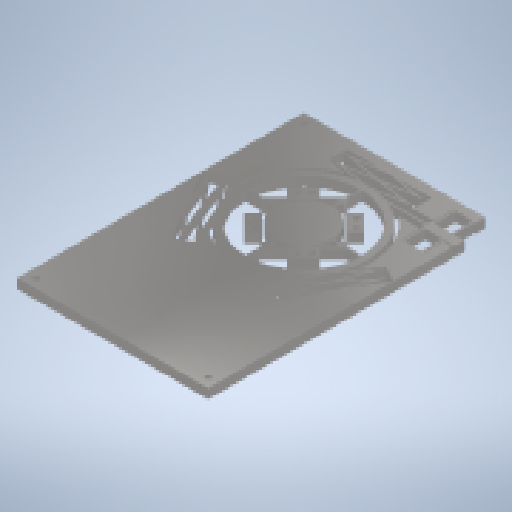
# Autodesk Inventor part: FlexBloc
Saved by Autodesk Inventor 2023 (Build 270158000, 158)
## iProperties
Created: 2023-03-17
Part Number: FlexBloc
Material: Steel, Mild
Document SubType Name: Modeling
Designer: Nathann
Density: 7.85 g/cm^3
Appearance: Semi-Polished
Mass: 505.648 g
Surface Area: 323.574 cm^2
Volume: 64.4137 cm^3
Author: Nathann
Autodesk Inventor part; units mm, degrees
ref_plane "YZ Plane" through (0, 0, 0) normal (1, 0, 0) x (0, 1, 0)
ref_plane "XZ Plane" through (0, 0, 0) normal (0, 1, 0) x (-1, 0, 0)
ref_plane "XY Plane" through (0, 0, 0) normal (0, 0, 1) x (1, 0, 0)
sketch "Sketch1" plane through (0, 0, 0) normal (0, 1, 0) x (-1, 0, 0)
  line L0 (0, 0) -> (100, 0)
  line L1 (100, 0) -> (100, 150)
  line L2 (100, 150) -> (0, 150)
  line L3 (0, 150) -> (0, 0)
  dimension "d0" = 150
  dimension "d1" = 100
  constraints: 8 end point, 2 parallel, 1 horizontal, 1 perpendicular
  measures "d0" distance of L2.end L0.start
  measures "d1" distance of L0.start L0.end
extrude "Extrusion1" add sketch "Sketch1" along normal blind 5
sketch "Sketch6" plane through (0, 5, 0) normal (0, 1, 0) x (1, 0, 0)
  circle A0 centre (-50, -50) radius 15
  line L0 (0, -150) -> (0, 0) projected
  line L1 (0, 0) -> (-100, 0) projected
  circle A1 centre (-50, -50) radius 30
  circle A2 centre (-50, -50) radius 33.541
  line L2 (-64.4545, -50.5) -> (-85.4944, -50.5)
  line L3 (-85.4944, -50.5) -> (-85.4944, -49.5)
  line L4 (-85.4944, -49.5) -> (-64.4545, -49.5)
  line L5 (-64.4545, -49.5) -> (-64.4545, -50.5)
  line L6 (-50, -50) -> (-59.276, -50)
  circle A3 centre (-50, -50) radius 36.041
  line L7 (-65, -50) -> (-80, -50)
  line L8 (-67.5, -50) -> (-70, -52.5)
  line L9 (-67.5, -50) -> (-70, -47.5)
  line L10 (-70, -52.5) -> (-70.7463, -51.7537)
  line L11 (-70, -47.5) -> (-74.2837, -51.7837)
  line L12 (-70, -52.5) -> (-72.5, -50)
  line L13 (-72.5, -50) -> (-70, -47.5)
  line L14 (-73.2071, -50) -> (-70.3536, -52.8536)
  line L15 (-70.3536, -52.8536) -> (-70, -52.5)
  line L16 (-73.2071, -50) -> (-70.3536, -47.1464)
  line L17 (-70.3536, -47.1464) -> (-70, -47.5)
  line L18 (-70.3536, -52.8536) -> (-65.8462, -57.3609)
  line L19 (-65.8462, -57.3609) -> (-65.1391, -56.6538)
  line L20 (-65.1391, -56.6538) -> (-69.6464, -52.1464)
  line L21 (-70.3536, -47.1464) -> (-65.8462, -42.6391)
  line L22 (-65.8462, -42.6391) -> (-65.1391, -43.3462)
  line L23 (-65.1391, -43.3462) -> (-69.6464, -47.8536)
  line L24 (-50, -50) -> (-54.8166, -54.8166)
  line L25 (-50, -50) -> (-57.7269, -42.2731)
  line L26 (-65.1391, -56.6538) -> (-70.0888, -61.6036)
  line L27 (-70.0888, -61.6036) -> (-65.8462, -65.8462)
  line L28 (-65.8462, -65.8462) -> (-60.8964, -60.8964)
  line L29 (-60.8964, -60.8964) -> (-65.1391, -56.6538)
  circle A4 centre (-65.8462, -61.6036) radius 1.5
  line L30 (-64.4545, -50) -> (-69.6304, -50)
  line L31 (-65.1391, -43.3462) -> (-70.0888, -38.3964)
  line L32 (-70.0888, -38.3964) -> (-65.8462, -34.1538)
  line L33 (-65.8462, -34.1538) -> (-60.8964, -39.1036)
  line L34 (-60.8964, -39.1036) -> (-65.1391, -43.3462)
  circle A5 centre (-65.8462, -38.3964) radius 1.5
  line L35 (-50, -64.4545) -> (-50, -69.6304)
  line L36 (-34.1538, -65.8462) -> (-39.1036, -60.8964)
  line L37 (-39.1036, -60.8964) -> (-43.3462, -65.1391)
  line L38 (-42.6391, -65.8462) -> (-43.3462, -65.1391)
  circle A6 centre (-38.3964, -65.8462) radius 1.5
  line L39 (-43.3462, -65.1391) -> (-38.3964, -70.0888)
  line L40 (-50, -67.5) -> (-52.5, -70)
  line L41 (-50, -67.5) -> (-47.5, -70)
  line L42 (-47.1464, -70.3536) -> (-42.6391, -65.8462)
  line L43 (-49.5, -64.4545) -> (-49.5, -85.4944)
  line L44 (-43.3462, -65.1391) -> (-47.8536, -69.6464)
  line L45 (-50.5, -85.4944) -> (-50.5, -64.4545)
  line L46 (-47.5, -70) -> (-48.2463, -70.7463)
  line L47 (-49.5, -85.4944) -> (-50.5, -85.4944)
  line L48 (-38.3964, -70.0888) -> (-34.1538, -65.8462)
  line L49 (-50.5, -64.4545) -> (-49.5, -64.4545)
  line L50 (-50, -65) -> (-50, -80)
  line L51 (-47.1464, -70.3536) -> (-47.5, -70)
  line L52 (-52.8536, -70.3536) -> (-52.5, -70)
  line L53 (-47.5, -70) -> (-50, -72.5)
  line L54 (-50, -73.2071) -> (-47.1464, -70.3536)
  line L55 (-50, -72.5) -> (-52.5, -70)
  line L56 (-50, -73.2071) -> (-52.8536, -70.3536)
  line L57 (-52.5, -70) -> (-48.2163, -74.2837)
  line L58 (-56.6538, -65.1391) -> (-52.1464, -69.6464)
  line L59 (-52.8536, -70.3536) -> (-57.3609, -65.8462)
  line L60 (-60.8964, -60.8964) -> (-56.6538, -65.1391)
  line L61 (-56.6538, -65.1391) -> (-61.6036, -70.0888)
  circle A7 centre (-61.6036, -65.8462) radius 1.5
  line L62 (-65.8462, -65.8462) -> (-60.8964, -60.8964)
  line L63 (-61.6036, -70.0888) -> (-65.8462, -65.8462)
  line L64 (-57.3609, -65.8462) -> (-56.6538, -65.1391)
  line L65 (-35.5455, -50) -> (-30.3696, -50)
  line L66 (-34.1538, -34.1538) -> (-39.1036, -39.1036)
  line L67 (-39.1036, -39.1036) -> (-34.8609, -43.3462)
  line L68 (-34.1538, -42.6391) -> (-34.8609, -43.3462)
  circle A8 centre (-34.1538, -38.3964) radius 1.5
  line L69 (-34.8609, -43.3462) -> (-29.9112, -38.3964)
  line L70 (-32.5, -50) -> (-30, -52.5)
  line L71 (-32.5, -50) -> (-30, -47.5)
  line L72 (-29.6464, -47.1464) -> (-34.1538, -42.6391)
  line L73 (-35.5455, -49.5) -> (-14.5056, -49.5)
  line L74 (-34.8609, -43.3462) -> (-30.3536, -47.8536)
  line L75 (-14.5056, -50.5) -> (-35.5455, -50.5)
  line L76 (-30, -47.5) -> (-29.2537, -48.2463)
  line L77 (-14.5056, -49.5) -> (-14.5056, -50.5)
  line L78 (-29.9112, -38.3964) -> (-34.1538, -34.1538)
  line L79 (-35.5455, -50.5) -> (-35.5455, -49.5)
  line L80 (-35, -50) -> (-20, -50)
  line L81 (-29.6464, -47.1464) -> (-30, -47.5)
  line L82 (-29.6464, -52.8536) -> (-30, -52.5)
  line L83 (-30, -47.5) -> (-27.5, -50)
  line L84 (-26.7929, -50) -> (-29.6464, -47.1464)
  line L85 (-27.5, -50) -> (-30, -52.5)
  line L86 (-26.7929, -50) -> (-29.6464, -52.8536)
  line L87 (-30, -52.5) -> (-25.7163, -48.2163)
  line L88 (-34.8609, -56.6538) -> (-30.3536, -52.1464)
  line L89 (-29.6464, -52.8536) -> (-34.1538, -57.3609)
  line L90 (-39.1036, -60.8964) -> (-34.8609, -56.6538)
  line L91 (-34.8609, -56.6538) -> (-29.9112, -61.6036)
  circle A9 centre (-34.1538, -61.6036) radius 1.5
  line L92 (-34.1538, -65.8462) -> (-39.1036, -60.8964)
  line L93 (-29.9112, -61.6036) -> (-34.1538, -65.8462)
  line L94 (-34.1538, -57.3609) -> (-34.8609, -56.6538)
  line L95 (-50, -35.5455) -> (-50, -30.3696)
  line L96 (-65.8462, -34.1538) -> (-60.8964, -39.1036)
  line L97 (-60.8964, -39.1036) -> (-56.6538, -34.8609)
  line L98 (-57.3609, -34.1538) -> (-56.6538, -34.8609)
  circle A10 centre (-61.6036, -34.1538) radius 1.5
  line L99 (-56.6538, -34.8609) -> (-61.6036, -29.9112)
  line L100 (-50, -32.5) -> (-47.5, -30)
  line L101 (-50, -32.5) -> (-52.5, -30)
  line L102 (-52.8536, -29.6464) -> (-57.3609, -34.1538)
  line L103 (-50.5, -35.5455) -> (-50.5, -14.5056)
  line L104 (-56.6538, -34.8609) -> (-52.1464, -30.3536)
  line L105 (-49.5, -14.5056) -> (-49.5, -35.5455)
  line L106 (-52.5, -30) -> (-51.7537, -29.2537)
  line L107 (-50.5, -14.5056) -> (-49.5, -14.5056)
  line L108 (-61.6036, -29.9112) -> (-65.8462, -34.1538)
  line L109 (-49.5, -35.5455) -> (-50.5, -35.5455)
  line L110 (-50, -35) -> (-50, -20)
  line L111 (-52.8536, -29.6464) -> (-52.5, -30)
  line L112 (-47.1464, -29.6464) -> (-47.5, -30)
  line L113 (-52.5, -30) -> (-50, -27.5)
  line L114 (-50, -26.7929) -> (-52.8536, -29.6464)
  line L115 (-50, -27.5) -> (-47.5, -30)
  line L116 (-50, -26.7929) -> (-47.1464, -29.6464)
  line L117 (-47.5, -30) -> (-51.7837, -25.7163)
  line L118 (-43.3462, -34.8609) -> (-47.8536, -30.3536)
  line L119 (-47.1464, -29.6464) -> (-42.6391, -34.1538)
  line L120 (-39.1036, -39.1036) -> (-43.3462, -34.8609)
  line L121 (-43.3462, -34.8609) -> (-38.3964, -29.9112)
  circle A11 centre (-38.3964, -34.1538) radius 1.5
  line L122 (-34.1538, -34.1538) -> (-39.1036, -39.1036)
  line L123 (-38.3964, -29.9112) -> (-34.1538, -34.1538)
  line L124 (-42.6391, -34.1538) -> (-43.3462, -34.8609)
  point P0 (-67.9675, -36.2751)
  point P1 (-63.7249, -67.9675)
  point P2 (-32.0325, -63.7249)
  point P3 (-36.2751, -32.0325)
  point P4 (-49.5, -72.7071)
  point P5 (-49.5, -79.9958)
  point P6 (-20.0042, -50.5)
  point P7 (-27.2929, -50.5)
  point P8 (-34.1538, -42.6391)
  point P9 (-27.2929, -49.5)
  point P10 (-20.0042, -49.5)
  point P11 (-49.5, -20.0042)
  point P12 (-49.5, -27.2929)
  point P13 (-68, -49.5)
  point P14 (-64.9917, -49.5)
  point P15 (-50.5, -35.0083)
  point P16 (-50.5, -32)
  point P17 (-49.5, -32)
  point P18 (-49.5, -35.0083)
  point P19 (-35.0083, -49.5)
  point P20 (-32, -49.5)
  point P21 (-32, -50.5)
  point P22 (-35.0083, -50.5)
  point P23 (-49.5, -64.9917)
  point P24 (-49.5, -68)
  point P25 (-50.5, -68)
  point P26 (-50.5, -64.9917)
  point P27 (-64.9917, -50.5)
  point P28 (-68, -50.5)
  point P29 (-57.3609, -34.1538)
  point P30 (-50.5, -27.2929)
  point P31 (-50.5, -20.0042)
  point P32 (-79.9958, -49.5)
  point P33 (-72.7071, -49.5)
  point P34 (-72.7071, -50.5)
  point P35 (-79.9958, -50.5)
  point P36 (-50.5, -79.9958)
  point P37 (-50.5, -72.7071)
  point P38 (-83.5373, -50.5)
  point P39 (-83.5373, -49.5)
  point P40 (-50.5, -16.4627)
  point P41 (-49.5, -16.4627)
  point P42 (-16.4627, -49.5)
  point P43 (-16.4627, -50.5)
  point P44 (-49.5, -83.5373)
  point P45 (-50.5, -83.5373)
  dimension "d80" = 30
  dimension "d81" = 60
  dimension "d78" = 50
  dimension "d79" = 50
  dimension "d82" = 67.082
  dimension "d83" = 0.5
  dimension "d84" = 0.5
  dimension "d91" = 72.082
  dimension "d92" = 5
  dimension "d93" = 2.5
  dimension "d94" = 2.5
  dimension "d95" = 45
  dimension "d96" = 45
  dimension "d97" = 0.5
  dimension "d98" = 0.5
  dimension "d99" = 0.5
  dimension "d100" = 45
  dimension "d101" = 45
  dimension "d102" = 6
  dimension "d103" = 7
  dimension "d104" = 3
  dimension "d105" = 3
  dimension "d106" = 3
  dimension "d107" = 3
  dimension "d108" = 7.5
  dimension "d109" = 3
  dimension "d110" = 6
  dimension "d111" = 7
  dimension "d112" = 3
  dimension "d113" = 3
  dimension "d114" = 3
  dimension "d117" = 360
  constraints: 246 end point, 20 point on line, 15 perpendicular, 10 centre point, 9 parallel, 3 coincident, 3 horizontal, 3 midpoint, 264 other
  measures "d78" distance from line of point (-50, -50) L0
  measures "d79" distance from line of L1 point (-50, -50)
  measures "d82" diameter of A2
  measures "d83" distance between parallel lines of L4 L6
  measures "d84" distance from line of point (-50, -50) L2
  measures "d91" diameter of A3
  measures "d92" distance of L8.start L12.end
  measures "d93" horizontal distance of L12.end L9.end
  measures "d94" horizontal distance of L8.end L12.end
  measures "d95" angle of L7 L8
  measures "d96" angle of L9 L7
  measures "d97" distance of L14.end L8.end
  measures "d98" distance between parallel lines of L10 L20
  measures "d99" distance between parallel lines of L23 L11
  measures "d100" angle of L24 L6
  measures "d101" angle of L25 L6
  measures "d102" distance of L28.end L19.end
  measures "d103" distance of L19.end L26.end
  measures "d104" distance from line of L27 A4.centre
  measures "d105" distance from line of L26 A4.centre
  measures "d106" diameter of A4
  measures "d107" distance from line of L24 A4.centre
  measures "d108" distance of L7.start L12.end
  measures "d109" distance of point (-67.968, -36.275) A5.centre
  measures "d110" distance of L33.end L22.end
  measures "d111" distance of L32.end L33.end
  measures "d112" distance from line of L33 A5.centre
  measures "d113" diameter of A5
  measures "d114" distance from line of A5.centre L25
extrude "Extrusion6" cut sketch "Sketch6" against normal blind 10 contours A0 L105 L100 L118 L120 L67 L74 L71 L73 | L75 L70 L88 L90 L37 L44 L41 L43 A0 | A0 L4 L9 L23 L34 L97 L104 L101 L103 | L84 L72 L69 L78 L123 L121 L119 L116 L105 A1 L73 | L45 L40 L58 L60 L29 L20 L8 L2 A0 | L75 A1 L43 L54 L42 L39 L48 L93 L91 L89 L86 | A2 L73 L77 L75 | L114 L102 L99 L108 L32 L31 L21 L16 L4 A1 L103 | A2 L103 L107 L105 | L45 A1 L2 L14 L18 L26 L27 L63 L61 L59 L56 | L43 L47 L45 A2 | A2 L2 L3 L4 | A4 | A5 | A6 | A7 | A8 | A9 | A10 | A11
sketch "Sketch7" plane through (0, 5, 0) normal (0, 1, 0) x (1, 0, 0)
  line L0 (-30.2515, -22) -> (6.5047, -22)
  line L1 (6.5047, -22) -> (6.5047, -15)
  line L2 (6.5047, -15) -> (-23.9617, -15)
  line L3 (-50, -60) -> (-28.7023, -38.7023)
  line L4 (-50, -60) -> (0, -60)
  line L5 (-11.682, -22) -> (-5.682, -22)
  line L6 (-2.365, -15) -> (-8.365, -15)
  line L7 (-5, -22) -> (-17, -22)
  line L8 (-17, -22) -> (-17, -32)
  line L9 (-17, -32) -> (-5, -32)
  line L10 (-5, -32) -> (-5, -22)
  line L11 (-5, -15) -> (-17, -15)
  line L12 (-17, -15) -> (-17, -5)
  line L13 (-17, -5) -> (-5, -5)
  line L14 (-5, -5) -> (-5, -15)
  line L15 (0, 0) -> (-100, 0) projected
  line L16 (0, -150) -> (0, 0) projected
  line L17 (-16.5, -32) -> (-15.5, -32)
  line L18 (-15.5, -32) -> (-15.5, -21)
  line L19 (-15.5, -21) -> (-16.5, -21)
  line L20 (-16.5, -21) -> (-16.5, -32)
  line L21 (-5.5, -32) -> (-6.5, -32)
  line L22 (-6.5, -32) -> (-6.5, -21)
  line L23 (-6.5, -21) -> (-5.5, -21)
  line L24 (-5.5, -21) -> (-5.5, -32)
  line L25 (-5.5, -5) -> (-6.5, -5)
  line L26 (-6.5, -5) -> (-6.5, -16)
  line L27 (-6.5, -16) -> (-5.5, -16)
  line L28 (-5.5, -16) -> (-5.5, -5)
  line L29 (-16.5, -5) -> (-15.5, -5)
  line L30 (-15.5, -5) -> (-15.5, -16)
  line L31 (-15.5, -16) -> (-16.5, -16)
  line L32 (-16.5, -16) -> (-16.5, -5)
  line L33 (-17.539, -21) -> (0, -21)
  line L34 (0, -21) -> (0, -16)
  line L35 (0, -16) -> (-17.539, -16)
  arc A0 (-49.5, -16.4627) -> (-50.5, -16.4627) centre (-50, -50) ccw projected
  line L36 (0, 0) -> (-5, 0)
  line L37 (-5, 0) -> (-5, -16)
  line L38 (-5, -16) -> (0, -16)
  line L39 (0, -16) -> (0, 0)
  line L40 (-17.539, -21) -> (-17.539, -16)
  line L41 (-20.9617, -19) -> (-17.539, -19)
  line L42 (-17.539, -19) -> (-17.539, -18)
  line L43 (-17.539, -18) -> (-20.9617, -18)
  line L44 (-23.9617, -15) -> (-23.9617, -22)
  line L45 (-23.9617, -22) -> (-30.2515, -22)
  line L46 (-20.9617, -18) -> (-20.9617, -19)
  point P0 (-5.5, -10.5)
  point P1 (-5, -27)
  point P2 (-16, -21)
  point P3 (-16, -16)
  point P4 (-17, -15)
  point P5 (-17, -22)
  point P6 (-15.5, -5)
  point P7 (-15.5, -16)
  point P8 (-6.5, -16)
  point P9 (-6.5, -5)
  point P10 (-5.5, -16)
  point P11 (0, -16)
  point P12 (0, -15)
  point P13 (0, -21)
  point P14 (0, -22)
  point P15 (-6.5, -32)
  point P16 (-5, -5)
  point P17 (-15.5, -15)
  point P18 (-16.5, -15)
  point P19 (-15.5, -22)
  point P20 (-16.5, -22)
  point P21 (-16.5, -15)
  point P22 (-16.5, -22)
  point P23 (-6.5, -22)
  point P24 (-15.5, -22)
  point P25 (-5.5, -22)
  point P26 (-5.5, -15)
  point P27 (-15.5, -15)
  point P28 (-6.5, -15)
  dimension "d125" = 45
  dimension "d128" = 10
  dimension "d133" = 12
  dimension "d134" = 12
  dimension "d135" = 5
  dimension "d136" = 1
  dimension "d137" = 1
  dimension "d138" = 1
  dimension "d139" = 1
  dimension "d140" = 0.5
  dimension "d141" = 0.5
  dimension "d142" = 11
  dimension "d144" = 11
  dimension "d145" = 11
  dimension "d146" = 10
  dimension "d147" = 11
  dimension "d164" = 5
  dimension "d169" = 0
  dimension "d170" = 5
  dimension "d171" = 1
  dimension "d172" = 2
  dimension "d202" = 5
  dimension "d214" = 3
  constraints: 90 end point, 17 parallel, 17 point on line, 13 horizontal, 12 perpendicular, 4 midpoint, 2 vertical
  measures "d125" angle of L3 L4
  measures "d128" distance of L9.end L7.start
  measures "d133" distance of L8.end L9.end
  measures "d134" distance of L12.end L13.end
  measures "d135" distance between parallel lines of L16 L10
  measures "d136" distance between parallel lines of L18 L20
  measures "d137" distance between parallel lines of L22 L24
  measures "d138" distance from line of L26 point (-5.5, -10.5)
  measures "d139" distance between parallel lines of L32 L30
  measures "d140" distance between parallel lines of L8 L20
  measures "d141" distance from line of point (-5, -27) L24
  measures "d142" distance of L17.end L18.end
  measures "d144" distance of L29.end L30.end
  measures "d145" distance of L27.end L25.start
  measures "d146" distance of L11.end L12.end
  measures "d147" distance of L21.end L22.end
  measures "d164" distance between parallel lines of L16 L37
  measures "d169" distance between parallel lines of L34 L16
  measures "d170" distance between parallel lines of L35 L33
  measures "d171" distance between parallel lines of L43 L41
  measures "d172" distance between parallel lines of L35 L43
  measures "d202" distance between parallel lines of L15 L13
  measures "d214" distance between parallel lines of L46 L44
extrude "Extrusion7" cut sketch "Sketch7" against normal blind 5 contours L44 L2 L32 L35 L40 L43 L46 L41 L33 L20 L0 | L0 L20 L9 L8 | L12 L13 L32 L2 | L18 L33 L22 L0 | L0 L22 L9 L18 | L30 L13 L26 L2 | L2 L26 L35 L30 | L24 L0 L10 L9 | L33 L16 L0 L24 | L16 L2 L1 L0 | L28 L13 L14 L2 | L2 L37 L35 L28 | L35 L37 L2 L16 | L14 L37 L15 L16 L2
sketch "Sketch9" plane through (0, 5, 0) normal (0, 1, 0) x (1, 0, 0)
  arc A0 (-35.0083, -49.5) -> (-49.5, -35.0083) centre (-50, -50) ccw projected
  line L0 (-50, -50) -> (-50, -7.3451)
  arc A1 (-49.5, -16.4627) -> (-50.5, -16.4627) centre (-50, -50) ccw projected
  line L1 (-50, -16.459) -> (-35, -13.959)
  line L2 (-35, -13.959) -> (-50, -11.459)
  line L3 (-50, -11.459) -> (-65, -13.959)
  line L4 (-65, -13.959) -> (-50, -16.459)
  line L5 (-50, -17.4728) -> (-28.9172, -13.959)
  line L6 (-28.9172, -13.959) -> (-50, -10.4452)
  line L7 (-50, -10.4452) -> (-71.0828, -13.959)
  line L8 (-71.0828, -13.959) -> (-50, -17.4728)
  line L9 (-28.9172, -13.959) -> (-71.0828, -13.959)
  line L10 (-65, -7.9452) -> (-50, -10.4452)
  line L11 (-71.0828, -7.9452) -> (-50, -11.459)
  line L12 (-50, -5.4452) -> (-65, -7.9452)
  line L13 (-50, -4.4314) -> (-71.0828, -7.9452)
  line L14 (-28.9172, -7.9452) -> (-71.0828, -7.9452)
  line L15 (-35, -7.9452) -> (-50, -5.4452)
  line L16 (-50, -11.459) -> (-28.9172, -7.9452)
  line L17 (-28.9172, -7.9452) -> (-50, -4.4314)
  line L18 (-50, -10.4452) -> (-35, -7.9452)
  arc A2 (-49.5, -16.4627) -> (-50.5, -16.4627) centre (-50, -50) ccw projected
  line L19 (-50, -50) -> (-50, -44.5788)
  line L20 (-57.3177, -17.267) -> (-72.0828, -14.8061)
  line L21 (-72.0828, -14.8061) -> (-72.0828, -5.2647)
  line L22 (-42.6823, -17.267) -> (-27.9172, -14.8061)
  line L23 (-27.9172, -14.8061) -> (-27.9172, -5.2647)
  line L24 (-23.9617, -15) -> (-17, -15) projected
  line L25 (-27.9172, -5.2647) -> (-45, -5.2647)
  line L26 (-55, -5.2647) -> (-72.0828, -5.2647)
  line L27 (-57.3177, -17.267) -> (-54.3685, -16.7447)
  line L28 (-42.6823, -17.267) -> (-45.6315, -16.7447)
  line L29 (-79.0474, -66.7705) -> (-88.7124, -55.0301)
  line L30 (-88.7124, -55.0301) -> (-83.3775, -69.2705)
  line L31 (-83.3775, -69.2705) -> (-73.7124, -81.0109)
  line L32 (-73.7124, -81.0109) -> (-79.0474, -66.7705)
  line L33 (-96.9619, -52.7692) -> (-75.8792, -89.2856)
  line L34 (-91.7538, -49.7623) -> (-70.6711, -86.2787)
  line L35 (-78.1694, -66.2636) -> (-91.7538, -49.7623)
  line L36 (-91.7538, -49.7623) -> (-84.2555, -69.7774)
  line L37 (-74.6888, -72.7038) -> (-76.6157, -70.4109)
  line L38 (-88.5856, -72.2774) -> (-78.9205, -84.0178)
  line L39 (-78.9205, -84.0178) -> (-84.2555, -69.7774)
  line L40 (-89.4636, -72.7843) -> (-75.8792, -89.2856)
  line L41 (-75.8792, -89.2856) -> (-83.3775, -69.2705)
  line L42 (-84.2555, -69.7774) -> (-70.6711, -86.2787)
  line L43 (-70.6711, -86.2787) -> (-78.1694, -66.2636)
  line L44 (-74.6888, -72.7038) -> (-69.4374, -86.7212)
  line L45 (-69.4374, -86.7212) -> (-77.7005, -91.4919)
  line L46 (-86.2419, -76.6978) -> (-77.7005, -91.4919)
  line L47 (-82.0065, -60.0292) -> (-80.9842, -62.8444)
  line L48 (-93.9205, -58.037) -> (-88.5856, -72.2774)
  line L49 (-96.9619, -52.7692) -> (-89.4636, -72.7843)
  line L50 (-83.3775, -69.2705) -> (-96.9619, -52.7692)
  line L51 (-99.7833, -53.2434) -> (-91.2419, -68.0375)
  line L52 (-91.5202, -48.4727) -> (-99.7833, -53.2434)
  line L53 (-82.0065, -60.0292) -> (-91.5202, -48.4727)
  line L54 (-84.2555, -69.7774) -> (-93.9205, -58.037)
  line L55 (-20.9526, -66.7705) -> (-26.2876, -81.0109)
  line L56 (-26.2876, -81.0109) -> (-16.6225, -69.2705)
  line L57 (-16.6225, -69.2705) -> (-11.2876, -55.0301)
  line L58 (-11.2876, -55.0301) -> (-20.9526, -66.7705)
  line L59 (-24.1208, -89.2856) -> (-3.0381, -52.7692)
  line L60 (-29.3289, -86.2787) -> (-8.2462, -49.7623)
  line L61 (-21.8306, -66.2636) -> (-29.3289, -86.2787)
  line L62 (-29.3289, -86.2787) -> (-15.7445, -69.7774)
  line L63 (-17.9935, -60.0292) -> (-19.0158, -62.8444)
  line L64 (-11.4144, -72.2774) -> (-6.0795, -58.037)
  line L65 (-6.0795, -58.037) -> (-15.7445, -69.7774)
  line L66 (-10.5364, -72.7843) -> (-3.0381, -52.7692)
  line L67 (-3.0381, -52.7692) -> (-16.6225, -69.2705)
  line L68 (-15.7445, -69.7774) -> (-8.2462, -49.7623)
  line L69 (-8.2462, -49.7623) -> (-21.8306, -66.2636)
  line L70 (-17.9935, -60.0292) -> (-8.4798, -48.4727)
  line L71 (-8.4798, -48.4727) -> (-0.2167, -53.2434)
  line L72 (-8.7581, -68.0375) -> (-0.2167, -53.2434)
  line L73 (-25.3112, -72.7038) -> (-23.3843, -70.4109)
  line L74 (-21.0795, -84.0178) -> (-11.4144, -72.2774)
  line L75 (-24.1208, -89.2856) -> (-10.5364, -72.7843)
  line L76 (-16.6225, -69.2705) -> (-24.1208, -89.2856)
  line L77 (-22.2995, -91.4919) -> (-13.7581, -76.6978)
  line L78 (-30.5626, -86.7212) -> (-22.2995, -91.4919)
  line L79 (-25.3112, -72.7038) -> (-30.5626, -86.7212)
  line L80 (-15.7445, -69.7774) -> (-21.0795, -84.0178)
  point P0 (0, 0)
  point P1 (-16.459, -50)
  point P2 (-16.459, -50)
  point P3 (-50, -1.3313)
  point P4 (-51, -4.2647)
  point P5 (-51, -4.5981)
  point P6 (-53.0414, -10.9521)
  point P7 (-46.9586, -10.9521)
  point P8 (-45.6315, -16.7447)
  point P9 (-51.4257, -26.4893)
  point P10 (-50, -26.459)
  point P11 (-42.6823, -17.267)
  point P12 (-57.3177, -17.267)
  point P13 (-88.8192, -73.567)
  point P14 (-89.1079, -73.7337)
  point P15 (-92.1483, -74.3344)
  point P16 (-86.9403, -71.3275)
  point P17 (-78.7941, -67.2017)
  point P18 (-69.648, -62.99)
  point P19 (-70.3871, -61.7705)
  point P20 (-79.2941, -66.3356)
  point P21 (-93.33, -44.9502)
  point P22 (-10.1808, -71.8349)
  point P23 (-9.8921, -72.0016)
  point P24 (-7.8517, -74.3344)
  point P25 (-13.0597, -71.3275)
  point P26 (-20.7059, -66.3356)
  point P27 (-28.9263, -60.5207)
  point P28 (-29.6129, -61.7705)
  point P29 (-21.2059, -67.2017)
  point P30 (-32.7082, -90.0498)
  point P31 (-85.3372, -66.89)
  point P32 (-82.2958, -72.1579)
  point P33 (-17.7042, -72.1579)
  point P34 (-14.6628, -66.89)
  dimension "d167" = 5
  dimension "d168" = 1
  dimension "d179" = 1
  dimension "d180" = 1
  dimension "d182" = 1.0138
  dimension "d185" = 6.0138
  dimension "d190" = 1
  dimension "d191" = 1
  dimension "d203" = 0
  dimension "d204" = 1
  dimension "d205" = 1
  dimension "d206" = 1
  dimension "d207" = 1
  dimension "d208" = 5
  dimension "d209" = 5
  dimension "d218" = 360
  constraints: 160 end point, 27 point on line, 5 equal length, 5 parallel, 3 vertical, 2 perpendicular, 1 horizontal, 207 other
  measures "d167" distance of L1.start L2.end
  measures "d168" distance between parallel lines of L5 L1
  measures "d179" distance between parallel lines of L8 L4
  measures "d180" distance between parallel lines of L7 L3
  measures "d182" distance of L5.start L1.start
  measures "d185" distance of L5.start L11.end
  measures "d190" horizontal distance of L13.start point (-51, -4.265)
  measures "d191" horizontal distance of point (-51, -4.598) L13.start
  measures "d203" distance between parallel lines of L19 L0
  measures "d204" distance between parallel lines of L8 L20
  measures "d205" distance between parallel lines of L5 L22
  measures "d206" distance from line of L5.end L23
  measures "d207" distance from line of L21 L7.end
  measures "d208" horizontal distance of L25.end L13.start
  measures "d209" horizontal distance of L13.start L26.start
extrude "Extrusion10" cut sketch "Sketch9" against normal blind 5 contours L4 L9 L0 | L0 L9 L1 | L5 L6 L16 L17 L25 L23 L22 L28 | L27 L20 L21 L26 L13 L11 L7 L8 | L9 L3 L0 | L0 L2 L9 | L10 L14 L0 | L0 L14 L18 | L14 L12 L15 | L32 L34 L29 | L34 L31 L30 | L36 L50 L49 L51 L52 L53 L47 L35 | L43 L37 L44 L45 L46 L40 L41 L42 | L39 L33 L54 | L38 L48 L33 | L58 L60 L55 | L60 L57 L56 | L62 L76 L75 L77 L78 L79 L73 L61 | L69 L63 L70 L71 L72 L66 L67 L68 | L65 L59 L80 | L64 L74 L59
sketch "Sketch11" plane through (0, 5, 0) normal (0, 1, 0) x (1, 0, 0)
  arc A0 (-64.9917, -50.5) -> (-50.5, -64.9917) centre (-50, -50) ccw projected
  line L0 (-91.5202, -48.4727) -> (-82.0065, -60.0292) projected
  circle A1 centre (-50, -50) radius 33.541
  line L1 (-49.5, -85.4944) -> (-49.5, -83.5373) projected
  line L2 (-70.6711, -86.2787) -> (-76.6157, -70.4109) projected
  line L3 (-23.3843, -70.4109) -> (-29.3289, -86.2787) projected
  line L4 (-8.2462, -49.7623) -> (-19.0158, -62.8444) projected
  line L5 (-45.6315, -16.7447) -> (-28.9172, -13.959) projected
  line L6 (-71.0828, -13.959) -> (-54.3685, -16.7447) projected
  arc A2 (-74.717, -75.4789) -> (-25.283, -75.4789) centre (-50, -50) ccw
  arc A3 (-15.5761, -58.6662) -> (-40.2932, -15.855) centre (-50, -50) ccw
  arc A4 (-59.7068, -15.855) -> (-84.8937, -56.5221) centre (-50, -50) ccw
  point P0 (0, 0)
  dimension "d220" = 67.082
  constraints: 7 point on circle, 6 point on line, 3 centre point, 2 coincident, 3 other
extrude "Extrusion11" cut sketch "Sketch11" against normal blind 5 contours A4 L6 A1 L0 | A1 L1 A2 L2 | L5 A3 L4 A1 | A1 L3 A2 L1
sketch "Sketch12" plane through (0, 5, 0) normal (0, 1, 0) x (1, 0, 0)
  line L0 (-17, -15) -> (-23.9617, -15) projected
  line L1 (-23.9617, -15) -> (-30.0605, -15)
  line L2 (-30.0605, -15) -> (-30.0605, -22)
  line L3 (-30.0605, -22) -> (-23.9617, -22)
  line L4 (-23.9617, -22) -> (-23.9617, -15)
  line L5 (-30.0605, -22) -> (-38.2015, -16.5201)
  line L6 (-38.2015, -16.5201) -> (-30.0605, -15)
  point P0 (0, 0)
  constraints: 12 end point, 2 parallel, 1 horizontal, 1 perpendicular
extrude "Extrusion12" cut sketch "Sketch12" against normal blind 5
sketch "Sketch13" plane through (0, 5, 0) normal (0, 1, 0) x (1, 0, 0)
  line L0 (-17.539, -18) -> (-20.9617, -18) projected
  line L1 (-20.9617, -18) -> (-41.4723, -18)
  line L2 (-41.4723, -18) -> (-41.4723, -19)
  line L3 (-41.4723, -19) -> (-20.9617, -19)
  line L4 (-20.9617, -19) -> (-20.9617, -18)
  point P0 (0, 0)
  constraints: 8 end point, 2 parallel, 1 horizontal, 1 perpendicular
extrude "Extrusion13" add sketch "Sketch13" against normal blind 5
sketch "Sketch14" plane through (0, 5, 0) normal (0, 1, 0) x (1, 0, 0)
  circle A0 centre (-95, -5) radius 1.5
  circle A1 centre (-95, -145) radius 1.5
  circle A2 centre (-5, -145) radius 1.5
  line L0 (0, -150) -> (0, -22) projected
  line L1 (-100, -150) -> (0, -150) projected
  line L2 (-100, 0) -> (-100, -150) projected
  line L3 (-5, 0) -> (-100, 0) projected
  point P0 (0, 0)
  dimension "d227" = 5
  dimension "d228" = 5
  dimension "d229" = 5
  dimension "d230" = 5
  dimension "d231" = 5
  dimension "d232" = 5
  dimension "d233" = 3
  dimension "d234" = 3
  dimension "d235" = 3
  constraints: 3 centre point
  measures "d227" distance from line of L0 A2.centre
  measures "d228" distance from line of L1 A2.centre
  measures "d229" distance from line of L1 A1.centre
  measures "d230" distance from line of L2 A1.centre
  measures "d231" distance from line of L3 A0.centre
  measures "d232" distance from line of L2 A0.centre
  measures "d233" diameter of A0
  measures "d234" diameter of A1
  measures "d235" diameter of A2
extrude "Extrusion14" cut sketch "Sketch14" against normal blind 5
equation "\"d2\" = woodThickness"
equation "\"d83\" = 0.5 * bladeThickness"
equation "\"d84\" = 0.5 * bladeThickness"
equation "\"d93\" = 0.5 * d92"
equation "\"d94\" = d93"
equation "\"d97\" = 0.5 * bladeThickness"
equation "\"d98\" = d97"
equation "\"d99\" = d98"
equation "\"d104\" = 0.5 * d102"
equation "\"d105\" = d104"
equation "\"d106\" = M3Hole"
equation "\"d107\" = d102 - d105"
equation "\"d109\" = d104"
equation "\"d110\" = d102"
equation "\"d111\" = d103"
equation "\"d112\" = d107"
equation "\"d113\" = d106"
equation "\"d114\" = d107"
equation "\"bladeThickness\" = 1"
equation "\"woodThickness\" = 5"
equation "\"bladeLenghtFlexRatio\" = 0.05"
equation "\"colRadius\" = 3"
equation "\"d14\" = bladeThickness"
equation "\"d16\" = d14"
equation "\"d19\" = d16"
equation "\"M3Hole\" = 3"
body "Solid1"
